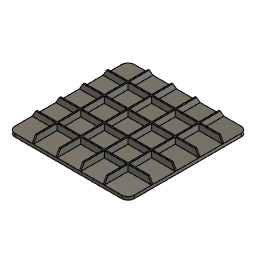
diffuser2 v8 (Autodesk Fusion 360 design; units mm, degrees)
Autodesk Fusion 360 part; units mm, degrees
note: some values were not read from the file. Chosen so that the rebuilt part matches the saved one: which bodies a step acts on. Set by a fixed rule: which sketch regions a step uses.
sketch "スケッチ1" plane through (0, 0, 0) normal (0, 1, 0) x (1, 0, 0)
  line L0 (1, 0) -> (18.2, 0)
  line L1 (19.2, -1) -> (19.2, -18.2)
  line L2 (18.2, -19.2) -> (1, -19.2)
  line L3 (0, -18.2) -> (0, -1)
  line L4 (3.8, -19.2) -> (3.8, 0)
  line L5 (4, -19.2) -> (4, 0)
  line L6 (7.6, 0) -> (7.6, -19.2)
  line L7 (7.8, -19.2) -> (7.8, 0)
  line L8 (19.2, -3.8) -> (0, -3.8)
  line L9 (0, -4) -> (19.2, -4)
  line L10 (19.2, -7.6) -> (0, -7.6)
  line L11 (0, -7.8) -> (19.2, -7.8)
  line L12 (0, -11.4) -> (19.2, -11.4)
  line L13 (19.2, -11.6) -> (0, -11.6)
  line L14 (0, -15.2) -> (19.2, -15.2)
  line L15 (19.2, -15.4) -> (0, -15.4)
  line L16 (11.4, -19.2) -> (11.4, 0)
  line L17 (11.6, 0) -> (11.6, -19.2)
  line L18 (15.2, -19.2) -> (15.2, 0)
  line L19 (15.4, 0) -> (15.4, -19.2)
  arc A0 (18.2, -19.2) -> (19.2, -18.2) centre (18.2, -18.2) ccw
  arc A1 (19.2, -1) -> (18.2, 0) centre (18.2, -1) ccw
  arc A2 (1, 0) -> (0, -1) centre (1, -1) ccw
  arc A3 (0, -18.2) -> (1, -19.2) centre (1, -18.2) ccw
  line L20 (-20.3302, 0) -> (25.6829, 0) construction
  line L21 (0, -22.3952) -> (0, 11.1848) construction
  dimension "d3" = 3.8
  dimension "d5" = 3.6
  dimension "d6" = 0.2
  dimension "d7" = 3.8
  dimension "d8" = 0.2
  dimension "d9" = 3.6
  dimension "d10" = 0.2
  dimension "d11" = 0.2
  dimension "d12" = 3.6
  dimension "d13" = 0.2
  dimension "d14" = 3.6
  dimension "d15" = 0.2
  dimension "d16" = 3.6
  dimension "d17" = 0.2
  dimension "d18" = 0.2
  dimension "d19" = 3.6
  dimension "d24" = 3.8
  dimension "d25" = 3.8
  dimension "d34" = 1
  constraint horizontal L0
  constraint vertical L1
  constraint horizontal L2
  constraint vertical L3
  constraint vertical L4
  constraint perpendicular L2 L5
  constraint perpendicular L2 L6
  constraint perpendicular L0 L7
  constraint perpendicular L3 L8
  constraint perpendicular L1 L9
  constraint perpendicular L3 L10
  constraint perpendicular L1 L11
  constraint coincident L2 L4.start
  constraint coincident L2 L5.start
  constraint coincident L2 L7.start
  constraint coincident L2 L6.end
  constraint coincident L0 L6.start
  constraint coincident L0 L4.end
  constraint coincident L3 L8.end
  constraint coincident L3 L11.start
  constraint coincident L1 L11.end
  constraint coincident L1 L10.start
  constraint coincident L1 L9.end
  constraint coincident L1 L8.start
  constraint coincident L3 L9.start
  constraint coincident L3 L10.end
  constraint coincident L3 L12.start
  constraint coincident L1 L12.end
  constraint perpendicular L1 L12
  constraint coincident L1 L13.start
  constraint coincident L3 L13.end
  constraint perpendicular L3 L13
  constraint coincident L3 L14.start
  constraint coincident L1 L14.end
  constraint perpendicular L1 L14
  constraint coincident L1 L15.start
  constraint coincident L3 L15.end
  constraint perpendicular L3 L15
  constraint coincident L2 L16.start
  constraint coincident L0 L16.end
  constraint perpendicular L0 L16
  constraint coincident L0 L17.start
  constraint coincident L2 L17.end
  constraint perpendicular L2 L17
  constraint coincident L2 L18.start
  constraint coincident L0 L18.end
  constraint perpendicular L0 L18
  constraint coincident L0 L19.start
  constraint coincident L2 L19.end
  constraint perpendicular L2 L19
  constraint tangent L1 A0
  constraint tangent L2 A0
  constraint tangent L0 A1
  constraint tangent L1 A1
  constraint equal A0 A1
  constraint tangent L0 A2
  constraint tangent L3 A2
  constraint equal A0 A2
  constraint tangent L2 A3
  constraint tangent L3 A3
  constraint equal A0 A3
  constraint perpendicular L3 L20
  constraint vertical L21
  constraint collinear L3 L21
  constraint collinear L0 L20
  measures "d3" distance of L0 L8
  measures "d5" distance of L9 L10
  measures "d6" distance of L10 L11
  measures "d7" distance of L3 L4
  measures "d8" distance of L4 L5
  measures "d9" distance of L5 L6
  measures "d10" distance of L6 L7
  measures "d11" distance of L8 L9
  measures "d12" distance of L7 L16
  measures "d13" distance of L16 L17
  measures "d14" distance of L17 L18
  measures "d15" distance of L18 L19
  measures "d16" distance of L11 L12
  measures "d17" distance of L12 L13
  measures "d18" distance of L14 L15
  measures "d19" distance of L13 L14
  measures "d24" distance of L1 L19
  measures "d25" distance of L2 L15
  measures "d34" radius of A0
extrude "押し出し1" add sketch "スケッチ1" along normal blind 0.5 contours L0 L3 L4 L8 A2 | L0 L5 L6 L8 | L3 L4 L9 L10 | L0 L7 L8 L16 | L5 L6 L9 L10 | L3 L4 L11 L12 | L0 L8 L17 L18 | L7 L9 L10 L16 | L5 L6 L11 L12 | L3 L4 L13 L14 | L0 L1 L8 L19 A1 | L9 L10 L17 L18 | L7 L11 L12 L16 | L5 L6 L13 L14 | L2 L3 L4 L15 A3 | L1 L9 L10 L19 | L11 L12 L17 L18 | L7 L13 L14 L16 | L2 L5 L6 L15 | L1 L11 L12 L19 | L13 L14 L17 L18 | L2 L7 L15 L16 | L1 L13 L14 L19 | L2 L15 L17 L18 | L1 L2 L15 L19 A0 makes body 1 at (14, 0, 14) makes body 2 at (17.9333, 0, 2.8667) makes body 3 at (9, 0, 2.5333) makes body 4 at (9, 0, 17.9333) makes body 5 at (5.2, 0, 5.2) makes body 6 at (1.2667, 0, 9) makes body 7 at (2.5333, 0, 14) makes body 8 at (6.4, 0, 1.2667) makes body 9 at (5.2, 0, 16.6667) makes body 10 at (9, 0, 5.2) makes body 11 at (16.6667, 0, 5.2) makes body 12 at (17.9333, 0, 14) makes body 13 at (12.8, 0, 17.9333) makes body 14 at (12.8, 0, 9) makes body 15 at (12.8, 0, 2.5333) makes body 16 at (10.2, 0, 14) makes body 17 at (5.2, 0, 9) makes body 18 at (1.2667, 0, 5.2) makes body 19 at (1.2667, 0, 16.3333) makes body 20 at (2.8667, 0, 1.2667) makes body 21 at (6.4, 0, 14) makes body 22 at (9, 0, 9) makes body 23 at (12.8, 0, 5.2) makes body 24 at (16.6667, 0, 9) makes body 25 at (17.9333, 0, 16.3333)
extrude "押し出し2" add sketch "スケッチ1" along normal blind 1.5 contours L0 L4 L5 L8 | L4 L5 L8 L9 | L3 L4 L8 L9 | L0 L6 L7 L8 | L5 L6 L8 L9 | L4 L5 L9 L10 | L6 L7 L8 L9 | L4 L5 L10 L11 | L3 L4 L10 L11 | L0 L8 L16 L17 | L7 L8 L9 L16 | L6 L7 L9 L10 | L5 L6 L10 L11 | L4 L5 L11 L12 | L8 L9 L16 L17 | L6 L7 L10 L11 | L4 L5 L12 L13 | L3 L4 L12 L13 | L0 L8 L18 L19 | L8 L9 L17 L18 | L9 L10 L16 L17 | L7 L10 L11 L16 | L6 L7 L11 L12 | L5 L6 L12 L13 | L4 L5 L13 L14 | L8 L9 L18 L19 | L10 L11 L16 L17 | L6 L7 L12 L13 | L4 L5 L14 L15 | L3 L4 L14 L15 | L1 L8 L9 L19 | L9 L10 L18 L19 | L10 L11 L17 L18 | L11 L12 L16 L17 | L7 L12 L13 L16 | L6 L7 L13 L14 | L5 L6 L14 L15 | L2 L4 L5 L15 | L10 L11 L18 L19 | L12 L13 L16 L17 | L6 L7 L14 L15 | L1 L10 L11 L19 | L11 L12 L18 L19 | L12 L13 L17 L18 | L13 L14 L16 L17 | L7 L14 L15 L16 | L2 L6 L7 L15 | L12 L13 L18 L19 | L14 L15 L16 L17 | L1 L12 L13 L19 | L13 L14 L18 L19 | L14 L15 L17 L18 | L2 L15 L16 L17 | L14 L15 L18 L19 | L1 L14 L15 L19 | L2 L15 L18 L19 bodies 1 2 3 4 5 6 7 8 9 10 11 12 13 14 15 16 17 18 19 20 21 22 23 24 25
sketch "スケッチ5" plane through (15.4, 0, 0) normal (1, 0, 0) x (0, 0, -1)
  line L0 (-19.2, 0.5) -> (-15.4, 0.5)
  line L1 (-15.4, 0.5) -> (-15.4, 1.5)
  line L2 (-15.4, 1.5) -> (-19.2, 1.5)
  line L3 (-19.2, 1.5) -> (-19.2, 0.5)
  line L4 (-19.2, 0.5) -> (-16.9184, 4.4518)
  line L5 (-16.9184, 4.4518) -> (-19.2, 4.4518)
  line L6 (-19.2, 4.4518) -> (-19.2, 0.5)
  dimension "d35" = 30
  constraint coincident L0.start L3.end
  constraint parallel L2 L5
  constraint perpendicular L2 L6
  measures "d35" angle of L4 L6
sketch "スケッチ6" plane through (15.4, 0, 0) normal (1, 0, 0) x (0, 0, -1)
  line L0 (-3.8, 0.5) -> (0, 0.5)
  line L1 (0, 0.5) -> (0, 1.5)
  line L2 (0, 1.5) -> (-3.8, 1.5)
  line L3 (-3.8, 1.5) -> (-3.8, 0.5)
  line L4 (0, 0.5) -> (0, 4.8319)
  line L5 (0, 4.8319) -> (-2.501, 4.8319)
  line L6 (-2.501, 4.8319) -> (0, 0.5)
  dimension "d36" = 30
  constraint coincident L0.end L1.start
  constraint perpendicular L0 L4
  constraint perpendicular L4 L5
  measures "d36" angle of L4 L6
extrude "押し出し5" cut sketch "スケッチ6" sketch "スケッチ5" against normal blind 14.5 contours L1 L2 L4 L6 of sketch 2 contours L2 L3 L4 L6 bodies 1
sketch "スケッチ3" plane through (0, 0, 15.4) normal (0, 0, 1) x (1, 0, 0)
  line L0 (0, 0.5) -> (3.8, 0.5)
  line L1 (3.8, 0.5) -> (3.8, 1.5)
  line L2 (3.8, 1.5) -> (0, 1.5)
  line L3 (0, 1.5) -> (0, 0.5)
  line L4 (0, 0.5) -> (0, 2.6672)
  line L5 (0, 2.6672) -> (1.2513, 2.6672)
  line L6 (1.2513, 2.6672) -> (0, 0.5)
  dimension "d30" = 30
  constraint coincident L0.start L3.end
  constraint perpendicular L2 L4
  constraint perpendicular L4 L5
  measures "d30" angle of L4 L6
sketch "スケッチ4" plane through (0, 0, 15.4) normal (0, 0, 1) x (1, 0, 0)
  line L0 (15.4, 0.5) -> (19.2, 0.5)
  line L1 (19.2, 0.5) -> (19.2, 1.5)
  line L2 (19.2, 1.5) -> (15.4, 1.5)
  line L3 (15.4, 1.5) -> (15.4, 0.5)
  line L4 (19.2, 0.5) -> (19.2, 2.9821)
  line L5 (19.2, 2.9821) -> (17.7669, 2.9821)
  line L6 (17.7669, 2.9821) -> (19.2, 0.5)
  dimension "d31" = 30
  constraint coincident L0.end L1.start
  constraint perpendicular L0 L4
  constraint perpendicular L4 L5
  measures "d31" angle of L4 L6
extrude "押し出し4" cut sketch "スケッチ3" sketch "スケッチ4" against normal blind 13 contours L2 L3 L4 L6 | L2 L4 L5 L6 of sketch 2 contours L1 L2 L4 L6 | L2 L4 L5 L6 bodies 1
